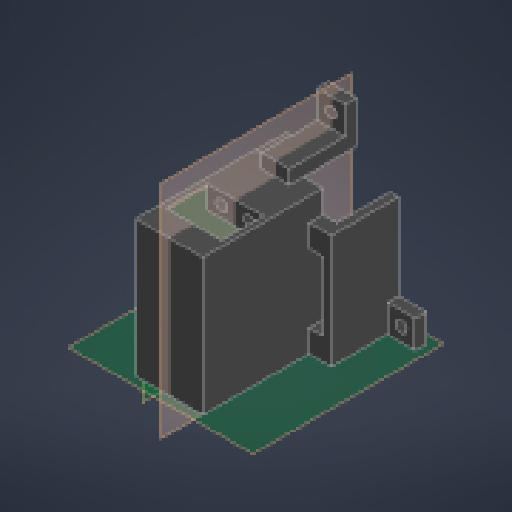
# Autodesk Inventor part: pitch_motor
Saved by Autodesk Inventor 2026.1 (Build 301233020, 233B)
## iProperties
Created: 2025-11-21
Part Number: pitch_motor
Material: 고무, 검은색
Document SubType Name: Modeling
Designer: jaewook
Density: 0.93 g/cm^3
Appearance: 고무 - 검은색
Author: jaewook
Autodesk Inventor part; units mm, degrees
ref_plane "YZ Plane" through (0, 0, 0) normal (1, 0, 0) x (0, 1, 0)
ref_plane "XZ Plane" through (0, 0, 0) normal (0, 1, 0) x (-1, 0, 0)
ref_plane "작업 평면1" through (-9.061, -9.3, 6.3) normal (-1, 0, 0) x (0, 1, 0)
sketch "스케치1" plane through (-9.061, -9.3, 6.3) normal (-1, 0, 0) x (0, 1, 0)
  line L0 (39.3939, -39.95) -> (-0.6061, -39.95)
  line L1 (-0.6061, 0.55) -> (39.3939, 0.55)
  line L2 (-0.6061, -12.65) -> (-7.8061, -12.65)
  line L3 (-7.8061, -12.65) -> (-7.8061, -9.45)
  line L4 (-7.8061, -9.45) -> (-0.6061, -9.45)
  line L5 (19.3939, -39.95) -> (19.3939, 0.55) construction
  line L6 (39.3939, -12.65) -> (46.5939, -12.65)
  line L7 (46.5939, -12.65) -> (46.5939, -9.45)
  line L8 (46.5939, -9.45) -> (39.3939, -9.45)
  line L9 (-0.6061, -39.95) -> (-0.6061, -12.65)
  line L10 (-0.6061, -9.45) -> (-0.6061, 0.55)
  line L11 (39.3939, 0.55) -> (39.3939, -9.45)
  line L12 (39.3939, -12.65) -> (39.3939, -39.95)
  line L13 (-9.1061, 1.1) -> (47.8939, 1.1)
  line L14 (39.6939, 1.1) -> (39.6939, -9.15)
  line L15 (39.6939, -9.15) -> (46.8939, -9.15)
  line L16 (46.8939, -9.15) -> (46.8939, -12.95)
  line L17 (46.8939, -12.95) -> (39.6939, -12.95)
  line L18 (39.6939, -12.95) -> (39.6939, -40.25)
  line L19 (39.6939, -40.25) -> (-0.9061, -40.25)
  line L20 (-0.9061, -40.25) -> (-0.9061, -12.95)
  line L21 (-0.9061, -12.95) -> (-8.1061, -12.95)
  line L22 (-8.1061, -12.95) -> (-8.1061, -9.15)
  line L23 (-8.1061, -9.15) -> (-0.9061, -9.15)
  line L24 (-0.9061, -9.15) -> (-0.9061, 1.1)
  line L25 (47.8939, 2.4305) -> (-9.1061, 2.4305)
  line L26 (-9.1061, 2.4305) -> (-9.1061, -41.8305)
  line L27 (-9.1061, -41.8305) -> (47.8939, -41.8305)
  line L28 (47.8939, -41.8305) -> (47.8939, 2.4305)
  line L29 (39.3939, -19.7) -> (-0.6061, -19.7) construction
  line L30 (39.6939, -26.25) -> (39.6939, -30.25)
  line L31 (-0.8061, 6.3) -> (19.1939, 6.3) projected
  line L32 (7.6194, 1.8) -> (13.6194, 1.8)
  line L33 (7.6194, 1.8) -> (13.6194, 1.8)
  line L34 (7.6194, 1.8) -> (13.6194, 1.8)
  line L35 (-0.9061, -31.1) -> (-4.9061, -31.1)
  line L36 (-4.9061, -31.1) -> (-4.9061, -36.1)
  line L37 (-4.9061, -36.1) -> (-0.9061, -36.1)
  line L38 (6.1939, 1.8) -> (12.1939, 1.8) projected
  point P0 (19.3939, -19.7)
  point P1 (9.1939, 6.3)
  dimension "d0" = 40.5
  dimension "d1" = 40
  dimension "d2" = 3.2
  dimension "d3" = 27.2
  dimension "d6" = 27.3
  dimension "d8" = 0.3
  dimension "d9" = 20.25
  dimension "d23" = 9.8
  dimension "d24" = 26
  dimension "d26" = 5
  dimension "d27" = 4
  dimension "d28" = 4.15
  constraints: 74 end point, 14 parallel, 9 perpendicular, 9 point on line, 4 horizontal, 4 midpoint, 4 symmetric about line, 2 collinear, 1 vertical, 12 other
  measures "d0" distance of L0.end L1.start
  measures "d1" distance of L0.start L0.end
  measures "d2" distance of L2.end L3.end
  measures "d3" distance between parallel lines of L3 L5
  measures "d6" distance between parallel lines of L0 L2
  measures "d8" distance between parallel lines of L10 L24
  measures "d9" distance between parallel lines of L29 L1
  measures "d23" distance from line of L10 point (9.194, 6.3)
  measures "d24" distance from line of L29 point (9.194, 6.3)
  measures "d26" distance of L35.end L36.end
  measures "d27" distance of L36.end L37.end
  measures "d28" distance between parallel lines of L19 L37
extrude "돌출1" add sketch "스케치1" against normal blind 22 contours L13 L24 L23 L22 L21 L20 L35 L36 L37 L19 L18 L17 L16 L15 L14 L28 L27 L26 | L20 L37 L36 L35
sketch "스케치4" plane through (12.939, -9.3, 6.3) normal (1, 0, 0) x (0, 0, -1)
  line L0 (-12.95, -0.9061) -> (-40.25, -0.9061) projected
  line L1 (-31.1, -0.9061) -> (-31.1, -4.9061) projected
  line L2 (-31.1, -4.9061) -> (-36.1, -4.9061) projected
  line L3 (-36.1, -4.9061) -> (-36.1, -0.9061) projected
  line L4 (-40.25, -0.9061) -> (-12.95, -0.9061) projected
  line L5 (-41.8305, -9.1061) -> (1.1, -9.1061) projected
  line L6 (-31.1, -4.9061) -> (-31.1, -9.1061)
  line L7 (-36.1, -4.9061) -> (-36.1, -9.1061)
  point P0 (6.3, 9.3)
  constraints: 4 end point, 2 perpendicular, 2 point on line
extrude "돌출4" cut sketch "스케치4" against normal blind 22
sketch "스케치2" plane through (-9.061, -9.3, 6.3) normal (-1, 0, 0) x (0, 0, 1)
  line L0 (-1.1, -0.9061) -> (-1.1, -9.1061) projected
  line L1 (-1.1, -9.1061) -> (41.8305, -9.1061) projected
  line L2 (41.8305, -9.1061) -> (41.8305, 47.8939) projected
  line L3 (41.8305, 47.8939) -> (-1.1, 47.8939) projected
  line L4 (-1.1, 47.8939) -> (-1.1, 39.6939) projected
  line L5 (-1.1, 47.8939) -> (41.8305, 47.8939)
  line L6 (41.8305, 47.8939) -> (41.8305, -9.1061)
  line L7 (41.8305, -9.1061) -> (-1.1, -9.1061)
  line L8 (-1.1, -9.1061) -> (-1.1, 47.8939)
  point P0 (-6.3, 9.3)
  point P1 (-1.1, -0.9061)
  constraints: 8 end point, 2 parallel, 1 horizontal, 1 perpendicular
extrude "돌출2" add sketch "스케치2" along normal blind 2
sketch "스케치3" plane through (12.939, -18.4061, 5.2) normal (0, 0, -1) x (-1, 0, 0)
  line L0 (22, 8.2) -> (0, 8.2) projected
  line L1 (22, 48.8) -> (0, 48.8) projected
  line L2 (22, 48.8) -> (22, 8.2) projected
  circle A0 centre (7.1, 4.2) radius 2
  line L3 (22, 28.5) -> (0, 28.5) construction
  line L4 (0, 8.2) -> (0, 48.8) projected
  circle A1 centre (7.1, 52.8) radius 2
  circle A2 centre (17, 4.2) radius 2
  circle A3 centre (17, 52.8) radius 2
  line L5 (12.05, 8.2) -> (12.05, 48.8)
  point P0 (12.939, 18.4061)
  dimension "d81" = 0
  dimension "d15" = 24.3
  dimension "d16" = 4
  dimension "d88" = 5
  dimension "d89" = 4.95
  dimension "d90" = 9.9
  constraints: 4 centre point, 4 end point, 2 equal radius, 2 midpoint, 2 point on line, 2 symmetric about line, 1 horizontal alignment, 1 perpendicular, 1 other
  measures "d15" distance from line of L3 A0.centre
  measures "d16" diameter of A0
  measures "d88" distance from line of A2.centre L2
  measures "d89" distance from line of L5 A2.centre
  measures "d90" distance of A1.centre A3.centre
extrude "돌출3" cut sketch "스케치3" against normal blind 40 contours A0 | A1 | A2 | A3
sketch "스케치5" plane through (12.939, -9.3, 6.3) normal (1, 0, 0) x (0, 0, -1)
  line L0 (1.1, -9.1061) -> (1.1, -0.9061) projected
  line L1 (-9.15, -0.9061) -> (-9.15, -8.1061) projected
  line L2 (-36.1, -9.1061) -> (-36.1, -0.9061) projected
  line L3 (-36.1, -0.9061) -> (-40.25, -0.9061) projected
  line L4 (-40.25, -0.9061) -> (-40.25, 39.6939) projected
  line L5 (-40.25, 39.6939) -> (-12.95, 39.6939) projected
  line L6 (-12.95, 39.6939) -> (-12.95, 46.8939) projected
  line L7 (-12.95, 46.8939) -> (-9.15, 46.8939) projected
  line L8 (-9.15, 46.8939) -> (-9.15, 39.6939) projected
  line L9 (-9.15, 39.6939) -> (1.1, 39.6939) projected
  line L10 (1.1, 39.6939) -> (1.1, 47.8939) projected
  line L11 (1.1, 47.8939) -> (-41.8305, 47.8939) projected
  line L12 (-41.8305, 47.8939) -> (-41.8305, -9.1061) projected
  line L13 (-41.8305, -9.1061) -> (-36.1, -9.1061) projected
  line L14 (-12.95, -8.1061) -> (-9.15, -8.1061) projected
  line L15 (-9.15, -8.1061) -> (1.1, -8.1061)
  line L16 (1.1, -8.1061) -> (1.1, 46.8939)
  line L17 (1.1, 46.8939) -> (-9.15, 46.8939)
  line L18 (-9.15, 46.8939) -> (-9.15, -8.1061)
  point P0 (6.3, 9.3)
  point P1 (-9.15, -0.9061)
  point P2 (1.1, -8.1061)
  point P3 (1.1, -0.9061)
  point P4 (1.1, 39.6939)
  point P5 (-9.15, 46.8939)
  constraints: 8 end point, 2 parallel, 1 horizontal, 1 perpendicular, 1 point on line
extrude "돌출5" cut sketch "스케치5" against normal up to surface (22 mm away) contours L15 L1 L18 L9 L16 L0 | L9 L8 L17 L10
sketch "스케치12" plane through (12.939, -10.2061, 46.55) normal (0, 0, -1) x (-1, 0, 0)
  line L0 (22, 40.6) -> (0, 40.6) projected
  line L1 (0, 0) -> (0, 40.6) projected
  line L2 (22, 47.8) -> (0, 47.8) projected
  line L3 (1.5, 48.8) -> (1.5, -8.2)
  line L4 (0, -8.2) -> (24, -8.2) projected
  line L5 (0, -7.2) -> (0, 0) projected
  line L6 (0, -8.2) -> (0, -7.2) projected
  line L7 (0, 40.6) -> (0, 47.8) projected
  line L8 (0, 48.8) -> (24, 48.8) projected
  line L9 (0, 47.8) -> (0, 48.8) projected
  point P0 (12.939, 10.2061)
  point P1 (1.5, 40.6)
  dimension "d55" = 1.5
  constraints: 2 end point, 2 point on line, 1 perpendicular
  measures "d55" distance between parallel lines of L5 L3
extrude "돌출12" add sketch "스케치12" along normal blind 41.35
sketch "스케치13" plane through (12.939, -18.4061, 5.2) normal (0, 0, -1) x (-1, 0, 0)
  line L0 (0, 0) -> (0, 57) projected
  line L1 (0, 0) -> (24, 0) projected
  line L2 (24, 57) -> (24, 0) projected
  line L3 (0, 57) -> (24, 57) projected
  line L4 (12, 0) -> (12, 57) construction
  line L5 (24, 28.5) -> (0, 28.5) construction
  line L6 (24, 8.2) -> (32, 8.2)
  line L7 (32, 8.2) -> (32, 16.2)
  line L8 (32, 16.2) -> (24, 16.2)
  line L9 (24, 16.2) -> (24, 8.2)
  line L10 (24, 40.8) -> (24, 48.8)
  line L11 (24, 0) -> (24, 57) projected
  line L12 (24, 48.8) -> (32, 48.8)
  line L13 (32, 48.8) -> (32, 40.8)
  line L14 (32, 40.8) -> (24, 40.8)
  line L15 (7, 57) -> (17, 57)
  line L16 (17, 57) -> (17, 62)
  line L17 (17, 62) -> (7, 62)
  line L18 (7, 62) -> (7, 57)
  point P0 (12.939, 18.4061)
  dimension "d70" = 8
  dimension "d71" = 8
  dimension "d72" = 8.2
  dimension "d73" = 10
  dimension "d74" = 5
  constraints: 28 end point, 4 midpoint, 4 parallel, 4 symmetric about line, 2 vertical alignment, 1 horizontal, 1 perpendicular, 1 point on line, 1 vertical, 1 other
  measures "d70" distance of L6.start L6.end
  measures "d71" distance of L6.end L7.end
  measures "d72" distance between parallel lines of L1 L6
  measures "d73" distance of L16.end L17.end
  measures "d74" distance of L15.end L16.end
extrude "돌출13" add sketch "스케치13" against normal blind 5 contours L18 L17 L16 L3 | L2 L8 L7 L6 | L2 L12 L13 L14
sketch "스케치14" plane through (-19.061, -10.2061, 5.2) normal (-1, 0, 0) x (0, 0, 1)
  line L0 (-34, 162.6) -> (-34, -37.7889) projected
  line L1 (-34, -37.7889) -> (-19, -37.7889) projected
  line L2 (-19, 162.6) -> (-19, -37.7889) projected
  line L3 (-34, 162.6) -> (-19, 162.6) projected
  line L4 (5, 0) -> (-19, 0)
  line L5 (-19, 0) -> (-19, 40.6)
  line L6 (-19, 40.6) -> (5, 40.6)
  line L7 (5, 40.6) -> (5, 0)
  line L8 (0, 32.6) -> (0, 40.6) projected
  line L9 (0, 32.6) -> (5, 32.6) projected
  line L10 (5, 40.6) -> (5, 32.6) projected
  line L11 (0, 40.6) -> (5, 40.6) projected
  point P0 (-5.2, 10.2061)
  point P1 (-19, 0)
  constraints: 8 end point, 2 parallel, 1 horizontal, 1 horizontal alignment, 1 perpendicular, 1 point on line
extrude "돌출14" add sketch "스케치14" against normal blind 3 contours L6 L8 L9 L7 L4 L2 | L6 L7 L9 L8
sketch "스케치15" plane through (-19.061, -10.2061, -13.8) normal (0, 0, -1) x (-1, 0, 0)
  line L0 (0, 40.6) -> (0, 0) projected
  line L1 (0, 0) -> (10, 0)
  line L2 (10, 0) -> (10, 10)
  line L3 (10, 10) -> (0, 10)
  line L4 (0, 10) -> (0, 0)
  point P0 (-19.061, 10.2061)
  point P1 (0, 10)
  dimension "d66" = 10
  dimension "d67" = 10
  constraints: 8 end point, 2 parallel, 1 horizontal, 1 perpendicular
  measures "d66" distance of L3.end L2.end
  measures "d67" distance of L2.end L1.end
extrude "돌출15" add sketch "스케치15" against normal blind 4
sketch "스케치16" plane through (12.939, -18.4061, 5.2) normal (0, 0, -1) x (-1, 0, 0)
  line L0 (17, 57) -> (17, 62) projected
  line L1 (17, 62) -> (7, 62) projected
  line L2 (7, 62) -> (7, 57) projected
  line L3 (7, 57) -> (17, 57) projected
  point P0 (12.939, 18.4061)
ref_plane "작업 평면2" through (-79.061, -70.6061, -13.8) normal (0, 0, 1) x (1, 0, 0)
extrude "돌출16" add sketch "스케치16" along normal up to surface (19 mm away)
sketch "스케치17" plane through (-4.061, 43.5939, 10.2) normal (0, 1, 0) x (1, 0, 0)
  line L0 (0, 0) -> (0, 24) projected
  line L1 (10, 24) -> (10, 0) projected
  line L2 (0, 24) -> (10, 24) projected
  line L3 (10, 20) -> (0, 20)
  point P0 (4.061, 10.2)
  dimension "d77" = 4
  constraints: 2 end point, 2 point on line, 1 perpendicular
  measures "d77" distance between parallel lines of L2 L3
extrude "돌출17" add sketch "스케치17" along normal blind 10
sketch "스케치18" plane through (-19.061, -10.2061, -9.8) normal (0, 0, 1) x (1, 0, 0)
  circle A0 centre (-5, 5) radius 2
  point P0 (19.061, 10.2061)
  dimension "d80" = 4
  constraints: 1 centre point
  measures "d80" diameter of A0
extrude "돌출18" cut sketch "스케치18" against normal through all
ref_plane "작업 평면3" through (0.939, -9.3, 6.3) normal (1, 0, 0) x (0, 0, -1)
sketch "스케치19" plane through (-4.061, 43.5939, -9.8) normal (0, 0, 1) x (1, 0, 0)
  line L0 (0, 10) -> (10, 10) projected
  line L1 (0, 0) -> (0, 10) projected
  circle A0 centre (5, 5) radius 2
  point P0 (4.061, -43.5939)
  dimension "d83" = 4
  dimension "d84" = 5
  dimension "d85" = 5
  constraints: 1 centre point
  measures "d83" diameter of A0
  measures "d84" distance from line of L1 A0.centre
  measures "d85" distance from line of L0 A0.centre
extrude "돌출19" cut sketch "스케치19" against normal through all
mirror "미러1" about plane through (0.939, -9.3, 6.3) normal (1, 0, 0) of "돌출13", "돌출14", "돌출15", "돌출18"
ref_plane "작업 평면4" through (20.939, -10.2061, 10.2) normal (0, -1, 0) x (1, 0, 0)
split "분할1" plane through (20.939, -10.2061, 10.2) removes the side toward (0, -1, 0)
sketch "스케치20" plane through (12.939, 38.5939, 48.1305) normal (0, 1, 0) x (1, 0, 0)
  line L0 (-22, 1.5805) -> (-22, 42.9305) projected
  line L1 (-22, 23.6445) -> (-2, 23.6445)
  line L2 (-2, 23.6445) -> (-2, 8.6445)
  line L3 (-2, 8.6445) -> (-22, 8.6445)
  line L4 (-22, 8.6445) -> (-22, 23.6445)
  point P0 (-12.939, 48.1305)
  point P1 (-22, 8.6445)
  dimension "d91" = 15
  dimension "d92" = 20
  constraints: 8 end point, 2 parallel, 1 horizontal, 1 perpendicular, 1 point on line
  measures "d91" distance of L1.end L2.end
  measures "d92" distance between parallel lines of L0 L2
extrude "돌출20" cut sketch "스케치20" against normal blind 10
